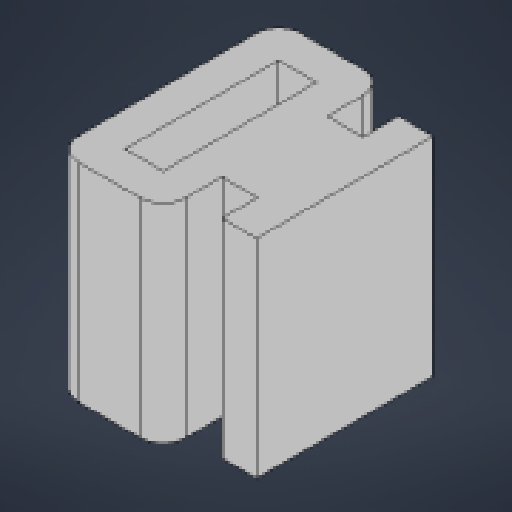
# Autodesk Inventor part: cajaIMU
Saved by Autodesk Inventor 2026.2 (Build 302298010, 298A)
## iProperties
Created: 2026-08-19
Part Number: cajaIMU
Material: Genérico
Document SubType Name: Modeling
Designer: samue
Density: 1 g/cm^3
Appearance: Valor por defecto
Author: samue
Autodesk Inventor part; units mm, degrees
ref_plane "YZ Plane" through (0, 0, 0) normal (1, 0, 0) x (0, 1, 0)
ref_plane "XZ Plane" through (0, 0, 0) normal (0, 1, 0) x (-1, 0, 0)
ref_plane "XY Plane" through (0, 0, 0) normal (0, 0, 1) x (1, 0, 0)
sketch "Boceto1" plane through (0, 0, 0) normal (0, 1, 0) x (-1, 0, 0)
  line L0 (0, 0) -> (-3.3, 0)
  line L1 (-3.3, 0) -> (-3.3, -13.3)
  line L2 (-3.3, -13.3) -> (0, -13.3)
  line L3 (0, -13.3) -> (0, 0)
  line L4 (3, 3) -> (-6.3, 3)
  line L5 (-6.3, 3) -> (-6.3, -16.3)
  line L6 (-6.3, -16.3) -> (3, -16.3)
  line L7 (3, -16.3) -> (3, 3)
  dimension "d0" = 3.3
  dimension "d1" = 13.3
  dimension "d2" = 3
  constraints: 16 end point, 4 parallel, 2 perpendicular, 1 horizontal, 3 other
  measures "d0" distance of L2.end L1.end
  measures "d1" distance of L1.end L0.end
  measures "d2" distance between parallel lines of L3 L7
extrude "Extrusión1" add sketch "Boceto1" along normal blind 15
fillet "Empalme1" radius 2 4 edges at (6.3, 7.5, 3) (-3, 7.5, 3) (-3, 7.5, -16.3) (6.3, 7.5, -16.3)
sketch "Boceto2" plane through (0, 0, 0) normal (0, -1, 0) x (1, 0, 0)
  line L0 (6.3, 1) -> (6.3, -14.3) projected
  arc A0 (6.3, 1) -> (4.3, 3) centre (4.3, 1) ccw projected
  line L1 (-1, 3) -> (4.3, 3) projected
  arc A1 (-1, 3) -> (-3, 1) centre (-1, 1) ccw projected
  line L2 (-3, -14.3) -> (-3, 1) projected
  arc A2 (-3, -14.3) -> (-1, -16.3) centre (-1, -14.3) ccw projected
  line L3 (4.3, -16.3) -> (-1, -16.3) projected
  arc A3 (4.3, -16.3) -> (6.3, -14.3) centre (4.3, -14.3) ccw projected
  point P0 (0, 0)
extrude "Extrusión2" add sketch "Boceto2" along normal blind 3
sketch "Boceto3" plane through (0, 15, 0) normal (0, 1, 0) x (1, 0, 0)
  line L0 (3.3, 13.3) -> (3.3, 0) projected
  line L1 (6.3, -1) -> (6.3, 14.3) projected
  line L2 (12.4, -1) -> (12.4, 14.3)
  line L3 (12.4, -1) -> (9.4, -1)
  line L4 (12.4, -1) -> (15.4, -1) construction
  line L5 (9.4, -1) -> (9.4, 2.1)
  line L6 (9.4, 2.1) -> (6.3, 2.1)
  line L7 (12.4, 14.3) -> (9.4, 14.3)
  line L8 (9.4, 14.3) -> (9.4, 11.2)
  line L9 (9.4, 11.2) -> (6.3, 11.2)
  point P0 (0, 0)
  dimension "d8" = 6.1
  dimension "d9" = 3
  dimension "d10" = 180
  dimension "d11" = 3.1
  dimension "d12" = 3.1
  constraints: 16 end point, 4 point on line, 3 perpendicular, 2 horizontal, 2 parallel, 1 collinear
  measures "d8" distance between parallel lines of L1 L2
  measures "d9" distance of L2.start L3.end
  measures "d10" angle of L3 L4
  measures "d11" distance of L3.end L5.end
  measures "d12" distance of L7.end L8.end
extrude "Extrusión3" add sketch "Boceto3" against normal up to surface (18 mm away)
sketch "Boceto4" plane through (0, -3, 0) normal (0, -1, 0) x (1, 0, 0)
  line L0 (3.3, -13.3) -> (3.3, 0) projected
  line L1 (3.3, 0) -> (0, 0) projected
  line L2 (0, 0) -> (0, -13.3) projected
  line L3 (0, -13.3) -> (3.3, -13.3) projected
  point P0 (1.65, -1.65)
  point P1 (1.65, -11.65)
  point P2 (1.65, -13.3)
  dimension "d15" = 1.65
  dimension "d16" = 1.65
  dimension "d17" = 1.65
  constraints: 1 midpoint
  measures "d15" distance from line of L0 point (1.65, -1.65)
  measures "d16" distance from line of L1 point (1.65, -1.65)
  measures "d17" distance of point (1.65, -13.3) point (1.65, -11.65)
hole "Agujero1" at (1.65, -3, -1.65) at (1.65, -3, -11.65) direction (0, 1, 0) diameter 3 end through all
